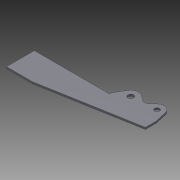
# Autodesk Inventor part: Plate
Saved by Autodesk Inventor 2014 (Build 180170000, 170)
## iProperties
Created: 2010-02-03
Part Number: Plate
Material: EN10025 P6 2004 S690QL
Document SubType Name: Modeling
Designer: stevew
Density: 7.86 g/cm^3
Mass: 23125 g
Surface Area: 4329.1 cm^2
Volume: 2942.12 cm^3
Description: 15 THK PLT
Appearance: Steel
Author: stevew
Revision Number: 2
Autodesk Inventor part; units mm, degrees
ref_plane "YZ Plane" through (0, 0, 0) normal (1, 0, 0) x (0, 1, 0)
ref_plane "XZ Plane" through (0, 0, 0) normal (0, 1, 0) x (-1, 0, 0)
ref_plane "XY Plane" through (0, 0, 0) normal (0, 0, 1) x (1, 0, 0)
sketch "Sketch2" plane through (0, 0, 0) normal (0, 0, 1) x (1, 0, 0)
  line L0 (0, 264) -> (0, -44) projected
  line L1 (-160, 0) -> (960, 0) projected
  line L2 (0, 0) -> (205, 0)
  line L3 (800, 220) -> (0, 220)
  line L4 (0, 220) -> (0, 0)
  line L5 (800, 104.9146) -> (800, 220)
  line L6 (205, 0) -> (800, 104.9146)
  dimension "d7" = 220
  dimension "d20" = 800
  dimension "d34" = 10
  dimension "d37" = 205
  constraints: 10 end point, 2 parallel, 2 point on line, 1 horizontal
  measures "d7" distance between parallel lines of L1 L3
  measures "d20" distance between parallel lines of L0 L5
  measures "d34" angle of L1 L6
  measures "d37" distance from line of L0 L2.end
extrude "Extrusion2" add sketch "Sketch2" along normal blind 15
sketch "Sketch5" plane through (0, 0, 0) normal (0, 0, -1) x (-1, 0, 0)
  line L0 (-800, 104.9146) -> (-800, 220) projected
  line L1 (-205, 0) -> (-800, 104.9146) projected
  line L2 (-800, 220) -> (-964, 220)
  line L3 (-964, 220) -> (-964, 133.8322)
  line L4 (-800, 104.9146) -> (-964, 133.8322)
  line L5 (0, 220) -> (0, 0) projected
  dimension "d40" = 964
  constraints: 6 end point, 2 perpendicular, 1 collinear
  measures "d40" distance between parallel lines of L5 L3
extrude "Extrusion4" add sketch "Sketch5" against normal up to surface (15 mm away)
sketch "Sketch3" plane through (0, 0, 0) normal (0, 0, -1) x (-1, 0, 0)
  line L0 (0, 220) -> (0, 0) projected
  line L1 (-800, 220) -> (0, 220) projected
  line L2 (-800, 104.9146) -> (-800, 220) projected
  line L3 (-595, 220) -> (-595, 240)
  circle A0 centre (-695, 288) radius 22.4
  circle A1 centre (-889, 301) radius 19.15
  arc A2 (-851.1955, 340.9477) -> (-942.6088, 313.2921) centre (-889, 301) ccw
  arc A3 (-643.9036, 319.4509) -> (-731.2075, 335.8437) centre (-695, 288) ccw
  line L4 (-595, 240) -> (-643.9036, 319.4509)
  line L5 (-942.6088, 313.2921) -> (-964, 220)
  line L6 (-964, 220) -> (-595, 220)
  line L7 (-731.2075, 335.8437) -> (-767.8616, 308.1042)
  line L8 (-851.1955, 340.9477) -> (-819.4942, 310.9471)
  arc A4 (-819.4942, 310.9471) -> (-767.8616, 308.1042) centre (-792, 340) ccw
  dimension "d23" = 44.8
  dimension "d26" = 695
  dimension "d28" = 68
  dimension "d29" = 20
  dimension "d35" = 100
  dimension "d41" = 38.3
  dimension "d42" = 81
  dimension "d43" = 194
  dimension "d45" = 110
  dimension "d46" = 60
  dimension "d47" = 97
  dimension "d48" = 40
  dimension "d49" = 120
  constraints: 12 end point, 6 point on circle, 6 tangent, 5 centre point, 2 coincident, 1 collinear, 1 parallel, 1 point on line
  measures "d23" diameter of A0
  measures "d26" distance from line of L0 A0.centre
  measures "d28" distance from line of L1 A0.centre
  measures "d29" distance of L3.start L3.end
  measures "d35" distance from line of L3 A0.centre
  measures "d41" diameter of A1
  measures "d42" distance from line of A1.centre L1
  measures "d43" horizontal distance of A1.centre A0.centre
  measures "d45" diameter of A2
  measures "d46" radius of A3
  measures "d47" horizontal distance of A0.centre A4.centre
  measures "d48" radius of A4
  measures "d49" distance from line of L6 A4.centre
extrude "Extrusion3" add sketch "Sketch3" against normal up to surface (15 mm away)
equation "\"d47\" = 0.5 * d43"
body "Solid1"
